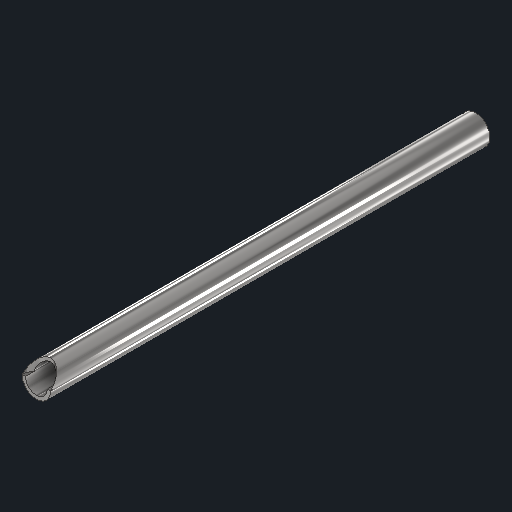
# Autodesk Inventor part: drive_shaft_center
Saved by Autodesk Inventor 2027.1 (Build 311270010, 270A)
## iProperties
Created: 2026-10-07
Part Number: drive_shaft_center
Material: Stainless Steel
Document SubType Name: Modeling
Designer: luca
Density: 8 g/cm^3
Appearance: Stahl - poliert
Author: luca
Autodesk Inventor part; units mm, degrees
ref_plane "YZ Plane" through (0, 0, 0) normal (1, 0, 0) x (0, 1, 0)
ref_plane "XZ Plane" through (0, 0, 0) normal (0, 1, 0) x (-1, 0, 0)
ref_plane "XY Plane" through (0, 0, 0) normal (0, 0, 1) x (1, 0, 0)
sketch "Skizze1" plane through (0, 0, 0) normal (0, 1, 0) x (-1, 0, 0)
  circle A0 centre (0, 0) radius 8.5
  circle A1 centre (0, 0) radius 6.5
  dimension "d0" = 17
  dimension "d1" = 13
  constraints: 2 centre point, 2 coincident
  measures "d0" diameter of A0
  measures "d1" diameter of A1
extrude "Extrusion1" add sketch "Skizze1" along normal blind 261
sketch "Sketch2" plane through (0, 0, 0) normal (0, 0, 1) x (1, 0, 0)
  line L0 (8.5, 261) -> (-8.5, 261) projected
  line L1 (8.5, 0) -> (-8.5, 0) projected
  circle A0 centre (0, 0) radius 8.5
  line L2 (-8.5, 0) -> (-8.5, 261) projected
  constraints: 1 centre point, 1 coincident, 1 tangent
extrude "Extrusion2" cut sketch "Sketch2" along normal blind 261 contours L1 A0 picked at (2.1208, 1.8788)
